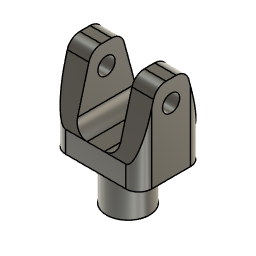
ujoint driveshaft v1 (Autodesk Fusion 360 design; units mm, degrees)
Autodesk Fusion 360 part; units mm, degrees
sketch "Sketch1" plane through (0, 0, 0) normal (0, 1, 0) x (1, 0, 0)
  line L0 (0, 0) -> (20, 0)
  line L1 (20, 0) -> (20, -20)
  line L2 (20, -20) -> (15, -20)
  line L3 (15, -20) -> (15, -5)
  line L4 (15, -5) -> (5, -5)
  line L5 (5, -5) -> (5, -20)
  line L6 (5, -20) -> (0, -20)
  line L7 (0, 0) -> (0, -20)
  dimension "d1" = 5
  dimension "d2" = 15
  dimension "d3" = 10
  constraint coincident L0.start L7.start
  constraint horizontal L0
  constraint perpendicular L0 L1
  constraint perpendicular L1 L2
  constraint perpendicular L2 L3
  constraint perpendicular L3 L4
  constraint perpendicular L4 L5
  constraint perpendicular L5 L6
  constraint perpendicular L0 L7
  measures "d1" distance of L1.end L2.end
  measures "d2" distance of L2.end L3.end
  measures "d3" distance of L3.end L4.end
extrude "Extrude1" add sketch "Sketch1" along normal blind 15
sketch "Sketch2" plane through (20, 0, 0) normal (1, 0, 0) x (0, 1, 0)
  line L0 (0, 20) -> (0, 0)
  line L1 (0, 0) -> (15, 0)
  line L2 (15, 0) -> (15, 20)
  line L3 (15, 20) -> (0, 20)
  line L4 (7.5, 20) -> (7.5, 15)
  circle A0 centre (7.5, 15) radius 2
  dimension "d6" = 5
  dimension "d7" = 4
  constraint midpoint L3 L4.start
  constraint perpendicular L3 L4
  constraint coincident L4.end A0.centre
  measures "d6" distance of L4.start L4.end
  measures "d7" diameter of A0
extrude "Extrude2" cut sketch "Sketch2" against normal through all contours A0
sketch "Sketch3" plane through (0, 0, 0) normal (0, 0, -1) x (1, 0, 0)
  line L0 (20, 0) -> (0, 0)
  line L1 (0, 0) -> (0, -15)
  line L2 (0, -15) -> (20, -15)
  line L3 (20, -15) -> (20, 0)
  line L4 (10, 0) -> (10, -7.5)
  circle A0 centre (10, -7.5) radius 5
  circle A1 centre (10, -7.5) radius 3
  dimension "d9" = 7.5
  dimension "d10" = 10
  dimension "d11" = 6
  constraint midpoint L0 L4.start
  constraint perpendicular L0 L4
  constraint coincident L4.end A0.centre
  constraint concentric A0 A1
  measures "d9" distance of L4.start L4.end
  measures "d10" diameter of A0
  measures "d11" diameter of A1
extrude "Extrude3" add sketch "Sketch3" along normal blind 10 contours A0
sketch "Sketch4" plane through (20, 0, 0) normal (1, 0, 0) x (0, 1, 0)
  circle A0 centre (7.5, 15) radius 2
  line L0 (0, 20) -> (0, 0)
  line L1 (0, 0) -> (15, 0)
  line L2 (15, 0) -> (15, 20)
  line L3 (15, 20) -> (0, 20)
  line L4 (0, 5) -> (4.0192, 20)
  line L5 (0, 5) -> (15, 5)
  line L6 (15, 5) -> (10.9808, 20)
  dimension "d14" = 75
  dimension "d15" = 75
  constraint coincident L0 L4.start
  constraint coincident L3 L4.end
  constraint coincident L2 L5.end
  constraint perpendicular L2 L5
  constraint coincident L3 L6.end
  measures "d14" angle of L4 L5
  measures "d15" angle of L5 L6
extrude "Extrude4" cut sketch "Sketch4" against normal through all contours L0 L3 L4 | L2 L3 L6
fillet "Fillet1" radius 3 4 edges at (2.5, 4.0192, 20) (2.5, 10.9808, 20) (17.5, 4.0192, 20) (17.5, 10.9808, 20)
fillet "Fillet2" radius 3 6 edges at (0, 0, 2.5) (20, 0, 2.5) (20, 15, 2.5) (5, 7.5, 5) (15, 7.5, 5) (0, 15, 2.5)
fillet "Fillet3" radius 1 1 edges at (5.3384, 5.6919, 0)
